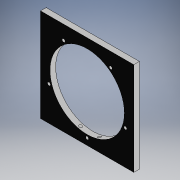
# Autodesk Inventor part: face_part
Saved by Autodesk Inventor 2019 (Build 230136000, 136)
## iProperties
Created: 2019-03-08
Part Number: face_part
Material: Generic
Document SubType Name: Modeling
Designer: Wilson Lab
Density: 1 g/cm^3
Appearance: Default
Author: Wilson Lab
Autodesk Inventor part; units mm, degrees
ref_plane "YZ Plane" through (0, 0, 0) normal (1, 0, 0) x (0, 1, 0)
ref_plane "XZ Plane" through (0, 0, 0) normal (0, 1, 0) x (-1, 0, 0)
ref_plane "XY Plane" through (0, 0, 0) normal (0, 0, 1) x (1, 0, 0)
sketch "Sketch1" plane through (0, 0, 0) normal (0, 0, 1) x (1, 0, 0)
  line L0 (-79, -79) -> (79, -79)
  line L1 (79, -79) -> (79, 79)
  line L2 (79, 79) -> (-79, 79)
  line L3 (-79, 79) -> (-79, -79)
  line L4 (-79, 0) -> (0, 0) construction
  line L5 (0, 0) -> (0, -79) construction
  point P0 (0, -79)
  dimension "d0" = 158
  dimension "d1" = 158
  constraints: 12 end point, 4 midpoint, 2 horizontal, 2 parallel, 2 perpendicular, 2 point on line
  measures "d0" distance of L1.end L2.end
  measures "d1" distance of L0.end L1.end
extrude "Extrusion1" add sketch "Sketch1" along normal blind 9.525
sketch "Sketch2" plane through (0, 0, 9.525) normal (0, 0, 1) x (1, 0, 0)
  circle A0 centre (0, 0) radius 68 construction
  line L0 (0, 0) -> (0, -68) construction
  circle A1 centre (0, 0) radius 68 construction
  circle A2 centre (0, 0) radius 68 construction
  circle A3 centre (0, 0) radius 68 construction
  circle A4 centre (0, 0) radius 68 construction
  point P0 (64.6718, -21.0132)
  point P1 (64.6718, -21.0132)
  point P2 (39.9694, 55.0132)
  point P3 (39.9694, 55.0132)
  point P4 (-39.9694, 55.0132)
  point P5 (-39.9694, 55.0132)
  point P6 (-64.6718, -21.0132)
  point P7 (-64.6718, -21.0132)
  dimension "d4" = 136
  dimension "d7" = 360
  constraints: 8 coincident, 2 end point, 1 vertical, 1 vertical alignment, 33 other
hole "Hole1" at (0, -68, 9.525) at (64.6718, -21.0132, 9.525) at (39.9694, 55.0132, 9.525) at (-39.9694, 55.0132, 9.525) at (-64.6718, -21.0132, 9.525) direction (0, 0, -1) diameter 5 end through all
sketch "Sketch4" plane through (0, 0, 9.525) normal (0, 0, 1) x (1, 0, 0)
  line L0 (79, -79) -> (79, 79) construction
  line L1 (79, 79) -> (-79, 79) construction
  line L2 (-79, 79) -> (-79, -79) construction
  line L3 (-79, -79) -> (79, -79) construction
  line L4 (-79, 0) -> (79, 0) construction
  line L5 (0, 79) -> (0, -79) construction
  circle A0 centre (0, 0) radius 63
  dimension "d16" = 126
  constraints: 4 end point, 4 midpoint, 1 centre point, 1 coincident
  measures "d16" diameter of A0
extrude "Extrusion2" cut sketch "Sketch4" against normal through all
sketch "Sketch5" plane through (-79, -79, 0) normal (0, -1, 0) x (1, 0, 0)
  line L0 (158, 0) -> (158, 9.525) construction
  line L1 (0, 9.525) -> (158, 9.525) construction
  line L2 (0, 0) -> (158, 0) construction
  line L3 (0, 0) -> (0, 9.525) construction
  line L4 (0, 4.7625) -> (158, 4.7625) construction
  point P0 (79, 0)
  point P1 (31.6, 4.7625)
  point P2 (126.4, 4.7625)
  point P3 (94.8, 4.7625)
  point P4 (63.2, 4.7625)
  dimension "d19" = 31.6
  dimension "d20" = 31.6
  dimension "d21" = 31.6
  dimension "d22" = 31.6
  dimension "d23" = 31.6
  constraints: 4 point on line, 2 end point, 2 midpoint
  measures "d19" distance from line of point (31.6, 4.762) L3
  measures "d20" distance of point (31.6, 4.762) point (63.2, 4.762)
  measures "d21" distance of point (94.8, 4.762) point (126.4, 4.762)
  measures "d22" distance from line of L0 point (126.4, 4.762)
  measures "d23" distance of point (63.2, 4.762) point (94.8, 4.762)
hole "Hole2" at (-47.4, -79, 4.7625) at (47.4, -79, 4.7625) at (15.8, -79, 4.7625) at (-15.8, -79, 4.7625) direction (0, 1, 0) diameter 4.978 depth 19.05 tip angle 118 thread size "1/4-20 UNC" class "2B" standard "ANSI Unified Screw Threads"
body "Solid1"
